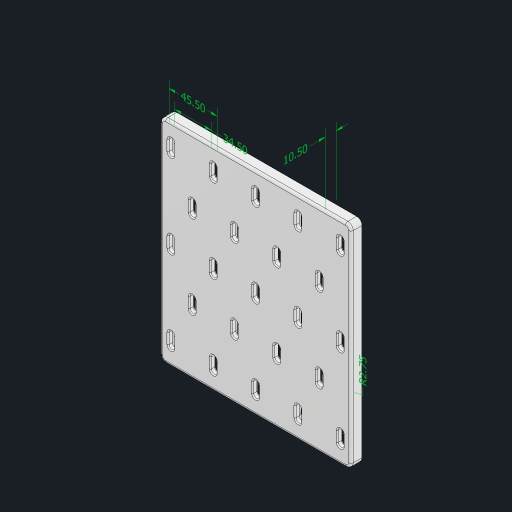
# Autodesk Inventor part: SKÅDIS Pegboard
Saved by Autodesk Inventor 2024 (Build 280153000, 153)
## iProperties
Created: 2024-02-06
Part Number: SKÅDIS Pegboard
Material: 일반
Document SubType Name: Modeling
Designer: KBU
Density: 1 g/cm^3
Appearance: 기본값
Author: KBU
Autodesk Inventor part; units mm, degrees
ref_plane "YZ Plane" through (0, 0, 0) normal (1, 0, 0) x (0, 1, 0)
ref_plane "XZ Plane" through (0, 0, 0) normal (0, 1, 0) x (-1, 0, 0)
ref_plane "XY Plane" through (0, 0, 0) normal (0, 0, 1) x (1, 0, 0)
sketch "스케치1" plane through (0, 0, 0) normal (0, 0, 1) x (1, 0, 0)
  line L0 (-110, -100) -> (110, -100)
  line L1 (110, -100) -> (110, 100)
  line L2 (110, 100) -> (-110, 100)
  line L3 (-110, 100) -> (-110, -100)
  line L4 (-110, -100) -> (110, 100) construction
  line L5 (110, -100) -> (-110, 100) construction
  line L6 (-100, 74) -> (-100, 84) construction
  line L7 (-102.75, 74) -> (-102.75, 84)
  line L8 (-97.25, 84) -> (-97.25, 74)
  arc A0 (-102.75, 74) -> (-97.25, 74) centre (-100, 74) ccw
  arc A1 (-97.25, 84) -> (-102.75, 84) centre (-100, 84) ccw
  line L9 (-62.75, 74) -> (-62.75, 84)
  line L10 (-60, 74) -> (-60, 84) construction
  line L11 (-57.25, 84) -> (-57.25, 74)
  arc A2 (-62.75, 74) -> (-57.25, 74) centre (-60, 74) ccw
  arc A3 (-57.25, 84) -> (-62.75, 84) centre (-60, 84) ccw
  line L12 (-22.75, 74) -> (-22.75, 84)
  line L13 (-20, 74) -> (-20, 84) construction
  line L14 (-17.25, 84) -> (-17.25, 74)
  arc A4 (-22.75, 74) -> (-17.25, 74) centre (-20, 74) ccw
  arc A5 (-17.25, 84) -> (-22.75, 84) centre (-20, 84) ccw
  line L15 (17.25, 74) -> (17.25, 84)
  line L16 (20, 74) -> (20, 84) construction
  line L17 (22.75, 84) -> (22.75, 74)
  arc A6 (17.25, 74) -> (22.75, 74) centre (20, 74) ccw
  arc A7 (22.75, 84) -> (17.25, 84) centre (20, 84) ccw
  line L18 (57.25, 74) -> (57.25, 84)
  line L19 (60, 74) -> (60, 84) construction
  line L20 (62.75, 84) -> (62.75, 74)
  arc A8 (57.25, 74) -> (62.75, 74) centre (60, 74) ccw
  arc A9 (62.75, 84) -> (57.25, 84) centre (60, 84) ccw
  line L21 (97.25, 74) -> (97.25, 84)
  line L22 (100, 74) -> (100, 84) construction
  line L23 (102.75, 84) -> (102.75, 74)
  arc A10 (97.25, 74) -> (102.75, 74) centre (100, 74) ccw
  arc A11 (102.75, 84) -> (97.25, 84) centre (100, 84) ccw
  line L24 (-80, 34.5) -> (-80, 44.5) construction
  line L25 (-77.25, 34.5) -> (-77.25, 44.5)
  line L26 (-82.75, 44.5) -> (-82.75, 34.5)
  arc A12 (-82.75, 34.5) -> (-77.25, 34.5) centre (-80, 34.5) ccw
  arc A13 (-77.25, 44.5) -> (-82.75, 44.5) centre (-80, 44.5) ccw
  arc A14 (-37.25, 44.5) -> (-42.75, 44.5) centre (-40, 44.5) ccw
  line L27 (-42.75, 44.5) -> (-42.75, 34.5)
  line L28 (-40, 34.5) -> (-40, 44.5) construction
  arc A15 (-42.75, 34.5) -> (-37.25, 34.5) centre (-40, 34.5) ccw
  line L29 (-37.25, 34.5) -> (-37.25, 44.5)
  arc A16 (2.75, 44.5) -> (-2.75, 44.5) centre (0, 44.5) ccw
  line L30 (-2.75, 44.5) -> (-2.75, 34.5)
  line L31 (0, 34.5) -> (0, 44.5) construction
  arc A17 (-2.75, 34.5) -> (2.75, 34.5) centre (0, 34.5) ccw
  line L32 (2.75, 34.5) -> (2.75, 44.5)
  arc A18 (42.75, 44.5) -> (37.25, 44.5) centre (40, 44.5) ccw
  line L33 (37.25, 44.5) -> (37.25, 34.5)
  line L34 (40, 34.5) -> (40, 44.5) construction
  arc A19 (37.25, 34.5) -> (42.75, 34.5) centre (40, 34.5) ccw
  line L35 (42.75, 34.5) -> (42.75, 44.5)
  arc A20 (82.75, 44.5) -> (77.25, 44.5) centre (80, 44.5) ccw
  line L36 (77.25, 44.5) -> (77.25, 34.5)
  line L37 (80, 34.5) -> (80, 44.5) construction
  arc A21 (77.25, 34.5) -> (82.75, 34.5) centre (80, 34.5) ccw
  line L38 (82.75, 34.5) -> (82.75, 44.5)
  line L39 (-100, -5) -> (-100, 5) construction
  line L40 (-102.75, -5) -> (-102.75, 5)
  arc A22 (-102.75, -5) -> (-97.25, -5) centre (-100, -5) ccw
  arc A23 (-97.25, 5) -> (-102.75, 5) centre (-100, 5) ccw
  line L41 (-97.25, 5) -> (-97.25, -5)
  line L42 (-62.75, -5) -> (-62.75, 5)
  line L43 (-60, -5) -> (-60, 5) construction
  arc A24 (-57.25, 5) -> (-62.75, 5) centre (-60, 5) ccw
  line L44 (-57.25, 5) -> (-57.25, -5)
  arc A25 (-62.75, -5) -> (-57.25, -5) centre (-60, -5) ccw
  line L45 (-22.75, -5) -> (-22.75, 5)
  line L46 (-20, -5) -> (-20, 5) construction
  line L47 (-17.25, 5) -> (-17.25, -5)
  arc A26 (-22.75, -5) -> (-17.25, -5) centre (-20, -5) ccw
  arc A27 (-17.25, 5) -> (-22.75, 5) centre (-20, 5) ccw
  line L48 (17.25, -5) -> (17.25, 5)
  line L49 (20, -5) -> (20, 5) construction
  arc A28 (17.25, -5) -> (22.75, -5) centre (20, -5) ccw
  line L50 (22.75, 5) -> (22.75, -5)
  arc A29 (22.75, 5) -> (17.25, 5) centre (20, 5) ccw
  line L51 (57.25, -5) -> (57.25, 5)
  line L52 (60, -5) -> (60, 5) construction
  line L53 (62.75, 5) -> (62.75, -5)
  arc A30 (57.25, -5) -> (62.75, -5) centre (60, -5) ccw
  arc A31 (62.75, 5) -> (57.25, 5) centre (60, 5) ccw
  line L54 (97.25, -5) -> (97.25, 5)
  line L55 (100, -5) -> (100, 5) construction
  arc A32 (97.25, -5) -> (102.75, -5) centre (100, -5) ccw
  line L56 (102.75, 5) -> (102.75, -5)
  arc A33 (102.75, 5) -> (97.25, 5) centre (100, 5) ccw
  line L57 (-100, -84) -> (-100, -74) construction
  line L58 (-102.75, -84) -> (-102.75, -74)
  arc A34 (-102.75, -84) -> (-97.25, -84) centre (-100, -84) ccw
  arc A35 (-97.25, -74) -> (-102.75, -74) centre (-100, -74) ccw
  line L59 (-97.25, -74) -> (-97.25, -84)
  line L60 (-62.75, -84) -> (-62.75, -74)
  line L61 (-60, -84) -> (-60, -74) construction
  arc A36 (-57.25, -74) -> (-62.75, -74) centre (-60, -74) ccw
  line L62 (-57.25, -74) -> (-57.25, -84)
  arc A37 (-62.75, -84) -> (-57.25, -84) centre (-60, -84) ccw
  line L63 (-22.75, -84) -> (-22.75, -74)
  line L64 (-20, -84) -> (-20, -74) construction
  line L65 (-17.25, -74) -> (-17.25, -84)
  arc A38 (-22.75, -84) -> (-17.25, -84) centre (-20, -84) ccw
  arc A39 (-17.25, -74) -> (-22.75, -74) centre (-20, -74) ccw
  line L66 (17.25, -84) -> (17.25, -74)
  line L67 (20, -84) -> (20, -74) construction
  arc A40 (17.25, -84) -> (22.75, -84) centre (20, -84) ccw
  line L68 (22.75, -74) -> (22.75, -84)
  arc A41 (22.75, -74) -> (17.25, -74) centre (20, -74) ccw
  line L69 (57.25, -84) -> (57.25, -74)
  line L70 (60, -84) -> (60, -74) construction
  line L71 (62.75, -74) -> (62.75, -84)
  arc A42 (57.25, -84) -> (62.75, -84) centre (60, -84) ccw
  arc A43 (62.75, -74) -> (57.25, -74) centre (60, -74) ccw
  line L72 (97.25, -84) -> (97.25, -74)
  line L73 (100, -84) -> (100, -74) construction
  arc A44 (97.25, -84) -> (102.75, -84) centre (100, -84) ccw
  line L74 (102.75, -74) -> (102.75, -84)
  arc A45 (102.75, -74) -> (97.25, -74) centre (100, -74) ccw
  line L75 (-80, -44.5) -> (-80, -34.5) construction
  line L76 (-77.25, -44.5) -> (-77.25, -34.5)
  arc A46 (-82.75, -44.5) -> (-77.25, -44.5) centre (-80, -44.5) ccw
  arc A47 (-77.25, -34.5) -> (-82.75, -34.5) centre (-80, -34.5) ccw
  line L77 (-82.75, -34.5) -> (-82.75, -44.5)
  arc A48 (2.75, -34.5) -> (-2.75, -34.5) centre (0, -34.5) ccw
  line L78 (2.75, -44.5) -> (2.75, -34.5)
  line L79 (0, -44.5) -> (0, -34.5) construction
  line L80 (-2.75, -34.5) -> (-2.75, -44.5)
  arc A49 (-2.75, -44.5) -> (2.75, -44.5) centre (0, -44.5) ccw
  arc A50 (42.75, -34.5) -> (37.25, -34.5) centre (40, -34.5) ccw
  line L81 (37.25, -34.5) -> (37.25, -44.5)
  line L82 (40, -44.5) -> (40, -34.5) construction
  line L83 (42.75, -44.5) -> (42.75, -34.5)
  arc A51 (37.25, -44.5) -> (42.75, -44.5) centre (40, -44.5) ccw
  arc A52 (82.75, -34.5) -> (77.25, -34.5) centre (80, -34.5) ccw
  line L84 (80, -44.5) -> (80, -34.5) construction
  line L85 (77.25, -34.5) -> (77.25, -44.5)
  arc A53 (77.25, -44.5) -> (82.75, -44.5) centre (80, -44.5) ccw
  line L86 (82.75, -44.5) -> (82.75, -34.5)
  arc A54 (-37.25, -34.5) -> (-42.75, -34.5) centre (-40, -34.5) ccw
  line L87 (-42.75, -34.5) -> (-42.75, -44.5)
  line L88 (-40, -44.5) -> (-40, -34.5) construction
  arc A55 (-42.75, -44.5) -> (-37.25, -44.5) centre (-40, -44.5) ccw
  line L89 (-37.25, -44.5) -> (-37.25, -34.5)
  line L90 (70, -100) -> (70, 100)
  point P0 (0, 0)
  point P1 (-100, 79)
  point P2 (-100, 71.25)
  point P3 (-100, 86.75)
  point P4 (-60, 79)
  point P5 (-60, 71.25)
  point P6 (-60, 86.75)
  point P7 (-20, 79)
  point P8 (-20, 71.25)
  point P9 (-20, 86.75)
  point P10 (20, 79)
  point P11 (20, 71.25)
  point P12 (20, 86.75)
  point P13 (60, 79)
  point P14 (60, 71.25)
  point P15 (60, 86.75)
  point P16 (100, 79)
  point P17 (100, 71.25)
  point P18 (100, 86.75)
  point P19 (100, 79)
  point P20 (-80, 39.5)
  point P21 (-80, 47.25)
  point P22 (-80, 31.75)
  point P23 (-40, 47.25)
  point P24 (-40, 39.5)
  point P25 (-40, 31.75)
  point P26 (0, 47.25)
  point P27 (0, 39.5)
  point P28 (0, 31.75)
  point P29 (40, 47.25)
  point P30 (40, 39.5)
  point P31 (40, 31.75)
  point P32 (80, 47.25)
  point P33 (80, 39.5)
  point P34 (80, 31.75)
  point P35 (-100, 0)
  point P36 (-100, -7.75)
  point P37 (-100, 7.75)
  point P38 (-60, 0)
  point P39 (-60, -7.75)
  point P40 (-60, 7.75)
  point P41 (-20, 0)
  point P42 (-20, -7.75)
  point P43 (-20, 7.75)
  point P44 (20, 0)
  point P45 (20, -7.75)
  point P46 (20, 7.75)
  point P47 (60, 0)
  point P48 (60, -7.75)
  point P49 (60, 7.75)
  point P50 (100, 0)
  point P51 (100, 0)
  point P52 (100, -7.75)
  point P53 (100, 7.75)
  point P54 (-100, -79)
  point P55 (-100, -86.75)
  point P56 (-100, -71.25)
  point P57 (-60, -79)
  point P58 (-60, -86.75)
  point P59 (-60, -71.25)
  point P60 (-20, -79)
  point P61 (-20, -86.75)
  point P62 (-20, -71.25)
  point P63 (20, -79)
  point P64 (20, -86.75)
  point P65 (20, -71.25)
  point P66 (60, -79)
  point P67 (60, -86.75)
  point P68 (60, -71.25)
  point P69 (100, -79)
  point P70 (100, -79)
  point P71 (100, -86.75)
  point P72 (100, -71.25)
  point P73 (-80, -39.5)
  point P74 (-80, -47.25)
  point P75 (-80, -31.75)
  point P76 (0, -31.75)
  point P77 (0, -39.5)
  point P78 (0, -47.25)
  point P79 (40, -31.75)
  point P80 (40, -39.5)
  point P81 (40, -47.25)
  point P82 (80, -31.75)
  point P83 (80, -39.5)
  point P84 (80, -47.25)
  point P85 (-40, -31.75)
  point P86 (-40, -39.5)
  point P87 (-40, -47.25)
  point P88 (100, -86.75)
  point P89 (-60, -86.75)
  point P90 (60, 79)
  dimension "d0" = 220
  dimension "d1" = 200
  dimension "d2" = 5.5
  dimension "d3" = 15.5
  dimension "d7" = 10
  dimension "d8" = 21
  dimension "d13" = 40
  dimension "d20" = 5.5
  dimension "d21" = 15.5
  dimension "d22" = 30
  dimension "d24" = 55
  dimension "d30" = 40
  dimension "d37" = 79
  dimension "d44" = 79
  dimension "d51" = 13.25
  dimension "d52" = 13.25
  dimension "d76" = 180
  dimension "d77" = 10
  constraints: 238 end point, 118 point on circle, 56 centre point, 8 tangent, 6 midpoint, 4 parallel, 4 vertical, 3 horizontal, 2 perpendicular, 2 point on line, 366 other
  measures "d0" distance of L1.end L2.end
  measures "d1" distance of L0.end L1.end
  measures "d2" distance between parallel lines of L8 L7
  measures "d3" distance of point (-100, 71.25) point (-100, 86.75)
  measures "d7" distance from line of point (-100, 79) L3
  measures "d8" distance from line of L2 point (-100, 79)
  measures "d13" distance of L7.start L9.start
  measures "d20" distance between parallel lines of L26 L25
  measures "d21" distance of point (-80, 47.25) point (-80, 31.75)
  measures "d22" distance from line of L3 point (-80, 39.5)
  measures "d24" vertical distance of point (-80, 31.75) point (-100, 86.75)
  measures "d30" distance of point (-80, 47.25) point (-40, 47.25)
  measures "d37" distance of point (-100, 79) point (-100, 0)
  measures "d44" distance of L24.start L75.start
  measures "d51" distance from line of L0 point (-60, -86.75)
  measures "d52" distance from line of L2 point (-100, 86.75)
  measures "d76" distance between parallel lines of L3 L90
  measures "d77" distance from line of L90 point (60, 79)
extrude "돌출1" add sketch "스케치1" along normal blind 5 contours L3 L2 L90 L0
sketch "스케치2" plane through (0, 0, 0) normal (0, 0, -1) x (-1, 0, 0)
  line L0 (-70, -100) -> (-70, 100) projected
  line L1 (110, -100) -> (-70, -100) projected
  line L2 (-70, 100) -> (110, 100)
  line L3 (110, 100) -> (110, -100)
  line L4 (110, -100) -> (-70, -100)
  line L5 (-70, -100) -> (-70, 100)
  line L6 (105, 95) -> (-65, 95)
  line L7 (-65, 95) -> (-65, -95)
  line L8 (-65, -95) -> (105, -95)
  line L9 (105, -95) -> (105, 95)
  line L10 (-12.5, 95) -> (-12.5, -95)
  line L11 (-17.25, -84) -> (-17.25, -74) projected
  line L12 (-7.5, -95) -> (-7.5, 95)
  line L13 (-2.75, -34.5) -> (-2.75, -44.5) projected
  line L14 (47.5, -95) -> (47.5, 95)
  line L15 (52.5, -95) -> (52.5, 95)
  line L16 (57.25, -74) -> (57.25, -84) projected
  line L17 (42.75, -44.5) -> (42.75, -34.5) projected
  point P0 (-2.75, -39.5)
  point P1 (57.25, -79)
  dimension "d79" = 5
  dimension "d80" = 4.75
  dimension "d81" = 4.75
  dimension "d82" = 5
  dimension "d83" = 4.75
  dimension "d84" = 4.75
  dimension "d85" = 5
  constraints: 24 end point, 6 point on line, 5 parallel, 5 perpendicular, 4 horizontal, 3 vertical, 2 midpoint, 8 other
  measures "d79" distance between parallel lines of L2 L6
  measures "d80" distance between parallel lines of L10 L11
  measures "d81" distance from line of L12 point (-2.75, -39.5)
  measures "d82" distance between parallel lines of L12 L10
  measures "d83" distance from line of point (57.25, -79) L15
  measures "d84" distance between parallel lines of L17 L14
  measures "d85" distance between parallel lines of L15 L14
extrude "돌출2" add sketch "스케치2" along normal blind 5.5 contours L0 L2 L3 L1 | L15 L8 L14 L6 | L12 L8 L10 L6
fillet "모깎기1" radius 5 4 edges at (-110, 100, -0.25) (70, -100, -0.25) (70, 100, -0.25) (-110, -100, -0.25)
fillet "모깎기2" radius 2.25 12 edges at (65, 95, -2.75) (12.5, 95, -2.75) (7.5, 95, -2.75) (-47.5, 95, -2.75) (-52.5, 95, -2.75) (-105, 95, -2.75) (-105, -95, -2.75) (-52.5, -95, -2.75) (-47.5, -95, -2.75) (7.5, -95, -2.75) (12.5, -95, -2.75) (65, -95, -2.75)
fillet "모깎기3" radius 1 184 edges at (-100, -86.75, 5) (-102.75, -79, 5) (-100, -71.25, 5) (-97.25, -79, 5) (-100, 71.25, 5) (-102.75, 79, 5) (-100, 86.75, 5) (-97.25, 79, 5) (-22.75, 79, 5) (-20, 86.75, 5) (-17.25, 79, 5) (-20, 71.25, 5) (-62.75, 79, 5) (-60, 86.75, 5) (-57.25, 79, 5) (-60, 71.25, 5) (17.25, 79, 5) (20, 86.75, 5) (22.75, 79, 5) (20, 71.25, 5) (57.25, 79, 5) (60, 86.75, 5) (62.75, 79, 5) (60, 71.25, 5) (37.25, 39.5, 5) (40, 47.25, 5) (42.75, 39.5, 5) (40, 31.75, 5) (-2.75, 39.5, 5) (0, 47.25, 5) (2.75, 39.5, 5) (0, 31.75, 5) (-40, 47.25, 5) (-37.25, 39.5, 5) (-40, 31.75, 5) (-42.75, 39.5, 5) (-82.75, 39.5, 5) (-80, 47.25, 5) (-77.25, 39.5, 5) (-80, 31.75, 5) (-100, -7.75, 5) (-102.75, 0, 5) (-100, 7.75, 5) (-97.25, 0, 5) (-60, -7.75, 5) (-62.75, 0, 5) (-60, 7.75, 5) (-57.25, 0, 5) (-20, 7.75, 5) (-17.25, 0, 5) (-20, -7.75, 5) (-22.75, 0, 5) (17.25, 0, 5) (20, 7.75, 5) (22.75, 0, 5) (20, -7.75, 5) (60, 7.75, 5) (62.75, 0, 5) (60, -7.75, 5) (57.25, 0, 5) (37.25, -39.5, 5) (40, -31.75, 5) (42.75, -39.5, 5) (40, -47.25, 5) (-2.75, -39.5, 5) (0, -31.75, 5) (2.75, -39.5, 5) (0, -47.25, 5) (-42.75, -39.5, 5) (-40, -31.75, 5) (-37.25, -39.5, 5) (-40, -47.25, 5) (-82.75, -39.5, 5) (-80, -31.75, 5) (-77.25, -39.5, 5) (-80, -47.25, 5) (-62.75, -79, 5) (-60, -71.25, 5) (-57.25, -79, 5) (-60, -86.75, 5) (-22.75, -79, 5) (-20, -71.25, 5) (-17.25, -79, 5) (-20, -86.75, 5) (17.25, -79, 5) (20, -71.25, 5) (22.75, -79, 5) (20, -86.75, 5) (57.25, -79, 5) (60, -71.25, 5) (62.75, -79, 5) (60, -86.75, 5) (57.25, 79, 0) (60, 86.75, 0) (62.75, 79, 0) (60, 71.25, 0) (20, 86.75, 0) (22.75, 79, 0) (20, 71.25, 0) (17.25, 79, 0) (-20, 71.25, 0) (-22.75, 79, 0) (-20, 86.75, 0) (-17.25, 79, 0) (-102.75, 79, 0) (-100, 86.75, 0) (-97.25, 79, 0) (-100, 71.25, 0) (-62.75, 79, 0) (-60, 86.75, 0) (-57.25, 79, 0) (-60, 71.25, 0) (-80, 31.75, 0) (-82.75, 39.5, 0) (-80, 47.25, 0) (-77.25, 39.5, 0) (-102.75, 0, 0) (-100, 7.75, 0) (-97.25, 0, 0) (-100, -7.75, 0) (-62.75, 0, 0) (-60, 7.75, 0) (-57.25, 0, 0) (-60, -7.75, 0) (-80, -31.75, 0) (-77.25, -39.5, 0) (-80, -47.25, 0) (-82.75, -39.5, 0) (-60, -71.25, 0) (-57.25, -79, 0) (-60, -86.75, 0) (-62.75, -79, 0) (-100, -86.75, 0) (-102.75, -79, 0) (-100, -71.25, 0) (-97.25, -79, 0) (-22.75, -79, 0) (-20, -71.25, 0) (-17.25, -79, 0) (-20, -86.75, 0) (20, -86.75, 0) (17.25, -79, 0) (20, -71.25, 0) (22.75, -79, 0) (40, -31.75, 0) (42.75, -39.5, 0) (40, -47.25, 0) (37.25, -39.5, 0) (0, -31.75, 0) (2.75, -39.5, 0) (0, -47.25, 0) (-2.75, -39.5, 0) (-40, -47.25, 0) (-42.75, -39.5, 0) (-40, -31.75, 0) (-37.25, -39.5, 0) (-20, 7.75, 0) (-17.25, 0, 0) (-20, -7.75, 0) (-22.75, 0, 0) (-40, 31.75, 0) (-42.75, 39.5, 0) (-40, 47.25, 0) (-37.25, 39.5, 0) (0, 31.75, 0) (-2.75, 39.5, 0) (0, 47.25, 0) (2.75, 39.5, 0) (40, 47.25, 0) (42.75, 39.5, 0) (40, 31.75, 0) (37.25, 39.5, 0) (22.75, 0, 0) (20, -7.75, 0) (17.25, 0, 0) (20, 7.75, 0) (60, 7.75, 0) (62.75, 0, 0) (60, -7.75, 0) (57.25, 0, 0) (60, -86.75, 0) (57.25, -79, 0) (60, -71.25, 0) (62.75, -79, 0)
fillet "모깎기4" radius 2.25 4 edges at (-20, -100, 5) (-20, 100, 5) (-108.5355, 98.5355, 5) (-110, 0, 5)
sketch "스케치5" plane through (0, 0, -5.5) normal (0, 0, -1) x (-1, 0, 0)
  line L0 (110, -95) -> (110, 95) projected
  line L1 (-70, 95) -> (-70, -95) projected
  line L2 (-7.5, -92.75) -> (-7.5, 92.75) projected
  line L3 (-70, -90.75) -> (110, -90.75)
  line L4 (110, -90.75) -> (110, -59.25)
  line L5 (110, -59.25) -> (-70, -59.25)
  line L6 (-70, -59.25) -> (-70, -90.75)
  line L7 (-70, -90.75) -> (110, -59.25) construction
  line L8 (110, -90.75) -> (-70, -59.25) construction
  arc A0 (16.25, -84) -> (23.75, -84) centre (20, -84) ccw projected
  arc A1 (23.75, -74) -> (16.25, -74) centre (20, -74) ccw projected
  circle A2 centre (-10, -69.25) radius 1.95
  circle A3 centre (-65, -64.25) radius 1.95
  circle A4 centre (-65, -95) radius 1.95
  circle A5 centre (-10, -90) radius 1.95
  line L9 (20, -111.2481) -> (20, -60.3206)
  circle A6 centre (50, -69.25) radius 1.95
  circle A7 centre (105, -64.25) radius 1.95
  circle A8 centre (105, -95) radius 1.95
  circle A9 centre (50, -90) radius 1.95
  line L10 (-65, -100) -> (105, -100) projected
  arc A10 (-63.75, -84) -> (-56.25, -84) centre (-60, -84) ccw projected
  arc A11 (-62.75, -84) -> (-57.25, -84) centre (-60, -84) ccw projected
  circle A12 centre (-10, -69.25) radius 3.5
  circle A13 centre (-10, -90) radius 3.5
  circle A14 centre (50, -69.25) radius 3.5
  circle A15 centre (50, -90) radius 3.5
  arc A16 (-70, -95) -> (-65, -100) centre (-65, -95) ccw projected
  line L11 (-14.75, -95) -> (-62.75, -95) projected
  circle A17 centre (-65, -64.25) radius 3.5
  circle A18 centre (-65, -95) radius 3.5
  circle A19 centre (105, -64.25) radius 3.5
  circle A20 centre (105, -95) radius 3.5
  point P0 (0, 0)
  point P1 (20, -75)
  point P2 (20, -87.75)
  point P3 (20, -70.25)
  point P4 (-60, -87.75)
  point P5 (-60, -86.75)
  dimension "d126" = 3
  dimension "d127" = 11
  dimension "d128" = 180
  dimension "d129" = 3.9
  dimension "d130" = 2.5
  dimension "d131" = 10
  dimension "d132" = 3.9
  dimension "d133" = 5
  dimension "d134" = 5
  dimension "d135" = 3.9
  dimension "d138" = 3.9
  dimension "d140" = 2.5
  dimension "d143" = 5
  dimension "d144" = 5
  dimension "d145" = 10
  dimension "d147" = 40.75
  dimension "d148" = 12.25
  dimension "d149" = 13.25
  dimension "d150" = 7
  dimension "d151" = 7
  dimension "d152" = 60
  dimension "d155" = 8.25
  dimension "d156" = 7
  dimension "d157" = 7
  constraints: 16 centre point, 14 end point, 8 symmetric about line, 4 coincident, 4 point on circle, 2 midpoint, 2 parallel, 1 horizontal, 1 perpendicular, 1 point on line, 1 vertical, 8 other
  measures "d126" distance from line of point (20, -87.75) L3
  measures "d127" distance from line of point (20, -70.25) L5
  measures "d128" distance of L4.end L5.end
  measures "d129" diameter of A2
  measures "d130" distance from line of L2 A2.centre
  measures "d131" distance from line of L5 A2.centre
  measures "d132" diameter of A3
  measures "d133" distance from line of L1 A3.centre
  measures "d134" distance from line of L5 A3.centre
  measures "d135" diameter of A4
  measures "d138" diameter of A5
  measures "d140" distance from line of L2 A5.centre
  measures "d143" distance of A4.centre L10.start
  measures "d144" distance from line of L1 A4.centre
  measures "d145" distance from line of L10 A5.centre
  measures "d147" distance between parallel lines of L10 L5
  measures "d148" distance from line of point (-60, -87.75) L10
  measures "d149" distance from line of L10 point (-60, -86.75)
  measures "d150" diameter of A12
  measures "d151" diameter of A13
  measures "d152" diameter of A2.centre L9
  measures "d155" distance from line of L11 point (-60, -86.75)
  measures "d156" diameter of A17
  measures "d157" diameter of A18
extrude "돌출7" cut sketch "스케치5" against normal blind 5 contours A9 L3 | L3 A9 | A5 L3 | L3 A5 | A2 | A3 | A4 | A6 | A7 | A8
extrude "돌출8" add sketch "스케치5" against normal up to surface (5.5 mm away) contours A15 L3 A9 | L3 A9 A15 | A12 L2 | L2 A12 | A13 L2 L3 | L3 L2 A13 | L2 L3 A5 A13 | L3 A5 L2 A13 | A14 | A17 | A18 | A19 | A20
fillet "모깎기11" radius 2 24 edges at (61.5, -95, -2.75) (65, -91.5, -2.75) (65, -60.75, -2.75) (65, -67.75, -2.75) (12.5, -92.4495, -2.75) (12.5, -87.5505, -2.75) (12.5, -66.8005, -2.75) (12.5, -71.6995, -2.75) (7.5, -92.4495, -2.75) (7.5, -87.5505, -2.75) (7.5, -66.8005, -2.75) (7.5, -71.6995, -2.75) (-47.5, -66.8005, -2.75) (-47.5, -71.6995, -2.75) (-47.5, -92.4495, -2.75) (-47.5, -87.5505, -2.75) (-105, -91.5, -2.75) (-105, -67.75, -2.75) (-105, -60.75, -2.75) (-101.5, -95, -2.75) (-52.5, -92.4495, -2.75) (-52.5, -87.5505, -2.75) (-52.5, -66.8005, -2.75) (-52.5, -71.6995, -2.75)
equation "\"d20\" = d2"
equation "\"d21\" = d3"
equation "\"d81\" = d80"
equation "\"d83\" = d80"
equation "\"d84\" = d80"
